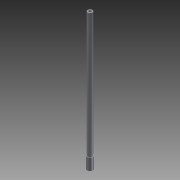
# Autodesk Inventor part: resonator
Saved by Autodesk Inventor 2012 (Build 160160000, 160)
## iProperties
Created: 2014-09-03
Part Number: resonator
Material: Default
Document SubType Name: Modeling
Designer: hannes.maierflaig
Density: 1 g/cm^3
Author: hannes.maierflaig
Autodesk Inventor part; units mm, degrees
ref_plane "YZ Plane" through (0, 0, 0) normal (1, 0, 0) x (0, 1, 0)
ref_plane "XZ Plane" through (0, 0, 0) normal (0, 1, 0) x (-1, 0, 0)
ref_plane "XY Plane" through (0, 0, 0) normal (0, 0, 1) x (1, 0, 0)
sketch "Skizze1" plane through (0, 0, 0) normal (0, 0, 1) x (1, 0, 0)
  circle A0 centre (0, 0) radius 4
  circle A1 centre (0, 0) radius 7.5
  dimension "d0" = 8
  dimension "d1" = 15
  constraints: 2 centre point, 2 coincident
  measures "d0" diameter of A0
  measures "d1" diameter of A1
extrude "Extrusion1" add sketch "Skizze1" along normal blind 400
sketch "Skizze2" plane through (0, 0, 0) normal (0, 0, -1) x (-1, 0, 0)
  circle A0 centre (0, 0) radius 7.5 projected
  circle A1 centre (0, 0) radius 2.5
  circle A2 centre (0, 0) radius 6
  circle A3 centre (0, 0) radius 9.065
  dimension "d4" = 5
  dimension "d5" = 12
  constraints: 3 centre point, 3 coincident
  measures "d4" diameter of A1
  measures "d5" diameter of A2
extrude "Extrusion2" add sketch "Skizze2" along normal blind 37 contours A0 | A2 | A3
